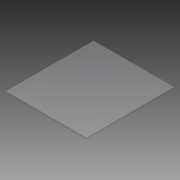
# Autodesk Inventor part: lid
Saved by Autodesk Inventor 2015 (Build 190159000, 159)
## iProperties
Created: 2015-10-15
Part Number: lid
Material: Polycarbonate, Clear
Description: insert part description/title
Document SubType Name: Modeling
Designer: c3132704
Density: 1.2 g/cm^3
Appearance: Polycarbonate - Clear
Author: c3132704
Part Category: insert part category here and press enter to fill value
Autodesk Inventor part; units mm, degrees
ref_plane "YZ Plane" through (0, 0, 0) normal (1, 0, 0) x (0, 1, 0)
ref_plane "XZ Plane" through (0, 0, 0) normal (0, 1, 0) x (-1, 0, 0)
ref_plane "XY Plane" through (0, 0, 0) normal (0, 0, 1) x (1, 0, 0)
sketch "Sketch1" plane through (0, 0, 0) normal (0, 0, 1) x (1, 0, 0)
  line L0 (0.9, 0) -> (0.9, 236.9272) construction
  line L1 (-2.4364, 238.4636) -> (-105.7636, 238.4636) construction
  line L2 (-105.7636, -1.5364) -> (-2.4364, -1.5364) construction
  line L3 (-219.1, 236.9272) -> (-219.1, 0) construction
  line L4 (1.9, 239.4636) -> (-220.1, 239.4636)
  line L5 (-220.1, 239.4636) -> (-220.1, -2.5364)
  line L6 (-220.1, -2.5364) -> (1.9, -2.5364)
  line L7 (1.9, -2.5364) -> (1.9, 239.4636)
  point P0 (0, 0)
  dimension "d0" = 1
  dimension "d1" = 1
  dimension "d2" = 1
  dimension "d3" = 1
  constraints: 8 end point, 2 parallel, 1 horizontal, 1 perpendicular
  measures "d0" distance between parallel lines of L0 L7
  measures "d1" distance between parallel lines of L2 L6
  measures "d2" distance between parallel lines of L5 L3
  measures "d3" distance between parallel lines of L1 L4
extrude "Extrusion1" add sketch "Sketch1" along normal blind 4
body "Solid1"
